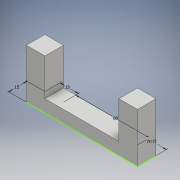
# Autodesk Inventor part: HandleR01
Saved by Autodesk Inventor 2018.1 (Build 221171000, 171)
## iProperties
Created: 2017-10-23
Part Number: HandleR01
Material: Generic
Document SubType Name: Modeling
Designer: s167968
Density: 1 g/cm^3
Appearance: Default
Author: s167968
Autodesk Inventor part; units mm, degrees
ref_plane "YZ Plane" through (0, 0, 0) normal (1, 0, 0) x (0, 1, 0)
ref_plane "XZ Plane" through (0, 0, 0) normal (0, 1, 0) x (-1, 0, 0)
ref_plane "XY Plane" through (0, 0, 0) normal (0, 0, 1) x (1, 0, 0)
sketch "Sketch3" plane through (0, 0, 0) normal (0, 0, 1) x (1, 0, 0)
  line L0 (-13.9172, 10.4459) -> (46.0828, 10.4459)
  line L1 (46.0828, 10.4459) -> (46.0828, -4.5541)
  line L2 (46.0828, -4.5541) -> (-13.9172, -4.5541)
  line L3 (-13.9172, -4.5541) -> (-13.9172, 10.4459)
  line L4 (46.0828, -4.5541) -> (61.0828, -4.5541)
  line L5 (61.0828, -4.5541) -> (61.0828, 10.4459)
  line L6 (61.0828, 10.4459) -> (46.0828, 10.4459)
  line L7 (46.0828, 10.4459) -> (46.0828, -4.5541)
  line L8 (-13.9172, 10.4459) -> (-28.9172, 10.4459)
  line L9 (-28.9172, 10.4459) -> (-28.9172, -4.5541)
  line L10 (-28.9172, -4.5541) -> (-13.9172, -4.5541)
  line L11 (-13.9172, -4.5541) -> (-13.9172, 10.4459)
  point P0 (0, 0)
  dimension "d0" = 15
  dimension "d1" = 15
  dimension "d2" = 15
  dimension "d3" = 60
  constraints: 24 end point, 6 parallel, 3 horizontal, 3 perpendicular, 2 point on line
  measures "d0" distance of L8.end L9.end
  measures "d1" distance of L0.start L8.end
  measures "d2" distance of L5.end L6.end
  measures "d3" distance of L0.start L0.end
extrude "Extrusion1" add sketch "Sketch3" along normal blind 10 contours L0 L1 L2 L3
extrude "Extrusion2" add sketch "Sketch3" along normal blind 40 contours L3 L10 L9 L8 | L6 L5 L4 L1
equation "\"d2\" = d1"
body "Solid1"
